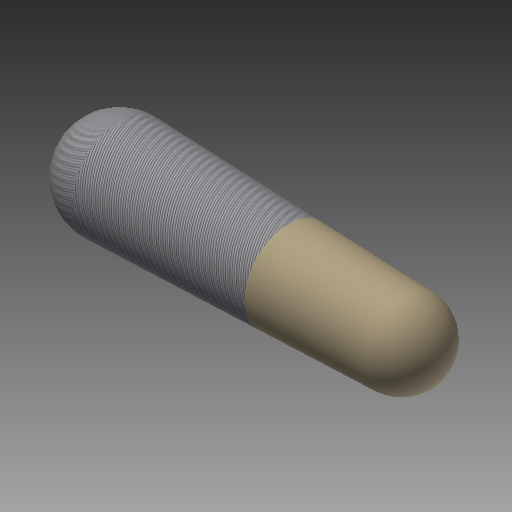
# Autodesk Inventor part: 3D HUMAN
Saved by Autodesk Inventor 2022 (Build 260153000, 153)
## iProperties
Category: PART
Part Number: 3D HUMAN
Document SubType Name: Modeling
Created: 2003-03-23
Designer: M.F.
Catalog Web Link: www.apollocanard.com
Density: 1 g/cm^3
Material: Generic
Appearance: Smooth - White
Control State: 0
Master: False
Checked Out: False
Shininess: 64.0
Length Units: 11272
Angle Units: 11279
Time Units: 11290
Mass Units: 11286
Length Display Precision: 3
Angle Display Precision: 2
Compacted: True
d1: 1.000 ul
d16: 10.300 in
d17: 3.640 in
d18: 2.980 in
d20: -6.180 in
Density: 0.0
Volumn: 0.0
Area: 0.0
PropertySet Name: Model Information
Title: iMandy
Author: M.F.
Autodesk Inventor part; units mm, degrees
ref_plane "YZ Plane" through (0, 0, 0) normal (1, 0, 0) x (0, 1, 0)
ref_plane "XZ Plane" through (0, 0, 0) normal (0, 1, 0) x (-1, 0, 0)
sketch "Sketch1" plane through (0, 0, 0) normal (0, 0, 1) x (1, 0, 0)
  circle A0 centre (0, 0) radius 46.228
  circle A1 centre (0, -261.62) radius 37.846
  line L0 (0, 46.228) -> (0, -299.466)
  line L1 (46.2043, -1.4811) -> (37.8266, -262.8325)
  dimension "d16" = 261.62
  dimension "d17" = 92.456
  dimension "d18" = 75.692
  constraints: 4 end point, 4 point on circle, 2 centre point, 2 tangent, 1 coincident, 1 point on line, 1 vertical, 1 vertical alignment
  measures "d16" distance of A1.centre A0.centre
  measures "d17" diameter of A0
  measures "d18" diameter of A1
revolve "Revolution1" add sketch "Sketch1" angle 360 about axis through (0, 46.228, 0) along (0, -1, 0) picked at (17.2426, 5.6008) picked at (12.6153, -261.62) contours A0 L0 | L1 A1 L0 A0 | A1 L0
ref_plane "Work Plane1" through (0, -156.972, 0) normal (0, 1, 0) x (-1, 0, 0)
split_face "Split1"
equation "\"d16\" = SHOULDER_TO_ELBOW"
equation "\"d17\" = SHOULDER_THK"
equation "\"d18\" = ELBOW_THK"
equation "\"d20\" = -0.6 * d16"
equation "\"SHOULDER_TO_ELBOW\" = 261.62"
equation "\"SHOULDER_THK\" = 92.456"
equation "\"ELBOW_THK\" = 75.692"
body "Solid1"
